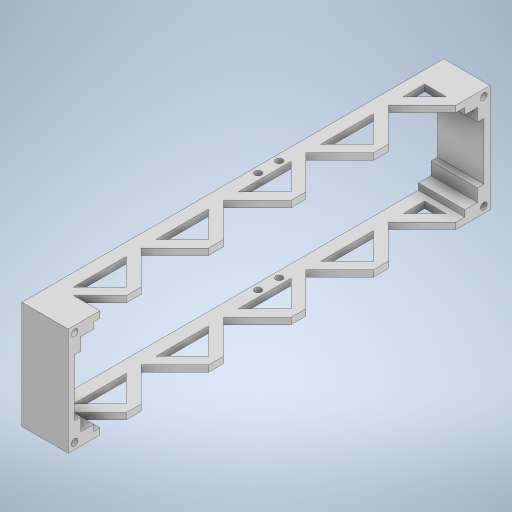
# Autodesk Inventor part: Middle_Bracket
Saved by Autodesk Inventor 2023 (Build 270158030, 158C)
## iProperties
Created: 2022-06-17
Part Number: Middle_Bracket
Material: Generic
Document SubType Name: Modeling
Designer: Mlees
Density: 1 g/cm^3
Appearance: Default
Author: Mlees
Autodesk Inventor part; units mm, degrees
ref_plane "YZ Plane" through (0, 0, 0) normal (1, 0, 0) x (0, 1, 0)
ref_plane "XZ Plane" through (0, 0, 0) normal (0, 1, 0) x (-1, 0, 0)
ref_plane "XY Plane" through (0, 0, 0) normal (0, 0, 1) x (1, 0, 0)
sketch "Sketch1" plane through (0, 0, 0) normal (1, 0, 0) x (0, 1, 0)
  line L0 (0, 0) -> (51, 0)
  line L1 (51, 0) -> (51, -200)
  line L2 (51, -200) -> (0, -200)
  line L3 (0, -200) -> (0, 0)
  line L4 (45, -6) -> (45, -12)
  line L5 (45, -12) -> (48, -12)
  line L6 (48, -12) -> (48, -188)
  line L7 (48, -188) -> (45, -188)
  line L8 (45, -194) -> (45, -188)
  line L9 (45, -12) -> (45, -6)
  line L10 (45, -6) -> (39, -6)
  line L11 (39, -6) -> (39, -3)
  line L12 (39, -3) -> (12, -3)
  line L13 (12, -3) -> (12, -6)
  line L14 (45, -6) -> (39, -6)
  line L15 (12, -6) -> (6, -6)
  line L16 (6, -6) -> (6, -12)
  line L17 (6, -12) -> (3, -12)
  line L18 (3, -12) -> (3, -188)
  line L19 (3, -188) -> (6, -188)
  line L20 (6, -6) -> (6, -12)
  line L21 (6, -188) -> (6, -194)
  line L22 (6, -194) -> (12, -194)
  line L23 (12, -194) -> (12, -197)
  line L24 (12, -197) -> (39, -197)
  line L25 (39, -197) -> (39, -194)
  line L26 (6, -194) -> (12, -194)
  line L27 (39, -194) -> (45, -194)
  circle A0 centre (48, -3) radius 1.625
  circle A1 centre (48, -197) radius 1.625
  circle A2 centre (3, -3) radius 1.625
  circle A3 centre (3, -197) radius 1.625
  dimension "d0" = 51
  dimension "d1" = 200
  dimension "d3" = 6
  dimension "d4" = 3
  dimension "d5" = 176
  dimension "d6" = 6
  dimension "d7" = 3
  dimension "d8" = 27
  dimension "d9" = 3
  constraints: 56 end point, 20 perpendicular, 14 parallel, 4 centre point, 1 horizontal
  measures "d0" distance of L1.end L2.end
  measures "d1" distance of L0.end L1.end
  measures "d3" distance of L4.start L4.end
  measures "d4" distance of L4.end L5.end
  measures "d5" distance of L5.end L6.end
  measures "d6" distance of L4.start L10.end
  measures "d7" distance of L10.end L11.end
  measures "d8" distance of L11.end L12.end
  measures "d9" distance of L16.end L17.end
extrude "Extrusion1" add sketch "Sketch1" along normal blind 44
sketch "Sketch2" plane through (0, 51, 0) normal (0, 1, 0) x (1, 0, 0)
  line L0 (0, 0) -> (44, 0) projected
  line L1 (44, 0) -> (44, 9)
  line L2 (44, 200) -> (44, 0) projected
  line L3 (44, 9) -> (44, 14)
  line L4 (0, 200) -> (0, 0) projected
  line L5 (44, 9) -> (0, 9)
  line L6 (0, 9) -> (0, 191)
  line L7 (0, 191) -> (44, 191)
  line L8 (44, 191) -> (44, 9)
  line L9 (9.5355, 15) -> (34.4645, 15)
  line L10 (38, 15) -> (83.2548, 15) construction
  line L11 (36.2322, 48.7678) -> (38, 50.5355)
  line L12 (7.7678, 48.7678) -> (6, 50.5355)
  line L13 (6, 43.4645) -> (6, 18.5355)
  line L14 (6, 18.5355) -> (18.4645, 31)
  line L15 (22, 34.5355) -> (36.2322, 48.7678)
  line L16 (34.4645, 15) -> (22, 27.4645)
  line L17 (18.4645, 31) -> (6, 43.4645)
  line L18 (9.5355, 15) -> (22, 27.4645)
  line L19 (25.5355, 31) -> (38, 43.4645)
  line L20 (38, 18.5355) -> (25.5355, 31)
  line L21 (22, 34.5355) -> (7.7678, 48.7678)
  line L22 (38, 18.5355) -> (38, 43.4645)
  line L23 (9.5355, 86.0711) -> (6, 89.6066)
  line L24 (34.4645, 86.0711) -> (38, 89.6066)
  line L25 (6, 82.5355) -> (6, 57.6066)
  line L26 (38, 57.6066) -> (38, 82.5355)
  line L27 (6, 50.5355) -> (22, 66.5355)
  line L28 (25.5355, 70.0711) -> (38, 82.5355)
  line L29 (38, 57.6066) -> (25.5355, 70.0711)
  line L30 (22, 73.6066) -> (9.5355, 86.0711)
  line L31 (6, 57.6066) -> (18.4645, 70.0711)
  line L32 (22, 73.6066) -> (34.4645, 86.0711)
  line L33 (38, 50.5355) -> (22, 66.5355)
  line L34 (18.4645, 70.0711) -> (6, 82.5355)
  line L35 (38, 89.6066) -> (83.2548, 89.6066) construction
  line L36 (9.5355, 125.1421) -> (6, 128.6777)
  line L37 (34.4645, 125.1421) -> (38, 128.6777)
  line L38 (6, 89.6066) -> (22, 105.6066)
  line L39 (25.5355, 109.1421) -> (38, 121.6066)
  line L40 (38, 89.6066) -> (22, 105.6066)
  line L41 (18.4645, 109.1421) -> (6, 121.6066)
  line L42 (6, 96.6777) -> (18.4645, 109.1421)
  line L43 (22, 112.6777) -> (34.4645, 125.1421)
  line L44 (38, 96.6777) -> (25.5355, 109.1421)
  line L45 (22, 112.6777) -> (9.5355, 125.1421)
  line L46 (38, 96.6777) -> (38, 121.6066)
  line L47 (6, 121.6066) -> (6, 96.6777)
  line L48 (38, 128.6777) -> (83.2548, 128.6777) construction
  line L49 (34.4645, 164.2132) -> (38, 167.7487)
  line L50 (9.5355, 164.2132) -> (6, 167.7487)
  line L51 (38, 135.7487) -> (38, 160.6777)
  line L52 (38, 174.8198) -> (38, 185)
  line L53 (38, 135.7487) -> (25.5355, 148.2132)
  line L54 (22, 151.7487) -> (9.5355, 164.2132)
  line L55 (6, 128.6777) -> (22, 144.6777)
  line L56 (25.5355, 148.2132) -> (38, 160.6777)
  line L57 (38, 128.6777) -> (22, 144.6777)
  line L58 (18.4645, 148.2132) -> (6, 160.6777)
  line L59 (6, 135.7487) -> (18.4645, 148.2132)
  line L60 (22, 151.7487) -> (34.4645, 164.2132)
  line L61 (6, 185) -> (6, 174.8198)
  line L62 (6, 160.6777) -> (6, 135.7487)
  line L63 (38, 167.7487) -> (22, 183.7487)
  line L64 (38, 167.7487) -> (62.397, 167.7487) construction
  line L65 (6, 167.7487) -> (22, 183.7487)
  line L66 (6, 167.7487) -> (30.397, 167.7487) construction
  line L67 (6, 174.8198) -> (16.1802, 185)
  line L68 (38, 174.8198) -> (27.8198, 185)
  line L69 (38, 185) -> (27.8198, 185)
  line L70 (16.1802, 185) -> (6, 185)
  dimension "d14" = 9
  dimension "d15" = 5
  dimension "d16" = 182
  dimension "d17" = 6
  dimension "d31" = 135
  dimension "d32" = 45
  dimension "d33" = 5
  dimension "d34" = 5
  constraints: 136 end point, 55 parallel, 14 perpendicular, 6 horizontal, 3 point on line
  measures "d14" distance of L0.end L1.end
  measures "d15" distance of L1.end L3.end
  measures "d16" distance of L5.end L6.end
  measures "d17" distance between parallel lines of L5 L9
  measures "d31" angle of L64 L63
  measures "d32" angle of L66 L65
  measures "d33" distance between parallel lines of L65 L67
  measures "d34" distance between parallel lines of L63 L68
extrude "Extrusion2" cut sketch "Sketch2" against normal through all contours L18 L16 L9 | L15 L21 L12 L27 L33 L11 | L17 L14 L13 | L19 L22 L20 | L23 L38 L40 L24 L32 L30 | L34 L31 L25 | L29 L28 L26 | L36 L55 L57 L37 L43 L45 | L39 L46 L44 | L42 L47 L41 | L60 L54 L50 L65 L63 L49 | L53 L56 L51 | L68 L69 L52 | L59 L62 L58 | L70 L67 L61
sketch "Sketch3" plane through (0, 51, 0) normal (0, 1, 0) x (1, 0, 0)
  line L0 (0, 200) -> (44, 200) projected
  line L1 (0, 188) -> (0, 12) projected
  line L2 (6, 121.6066) -> (6, 96.6777) projected
  point P0 (0, 0)
  point P1 (3, 109)
  point P2 (3, 119)
hole "Hole1" at (3, 51, -109) at (3, 51, -119) direction (0, -1, 0) diameter 3.25 depth 51 tip angle 118
sketch "Sketch4" plane through (0, 0, 0) normal (0, 0, 1) x (1, 0, 0)
  line L0 (38, 0) -> (22, 0) projected
  line L1 (0, 51) -> (44, 51) projected
  line L2 (22, 0) -> (44, 0)
  line L3 (44, 0) -> (44, 51)
  line L4 (44, 51) -> (22, 51)
  line L5 (22, 51) -> (22, 0)
  point P0 (0, 0)
  constraints: 8 end point, 2 parallel, 1 horizontal, 1 perpendicular
extrude "Extrusion3" cut sketch "Sketch4" against normal up to surface (200 mm away)
body "Solid1"
